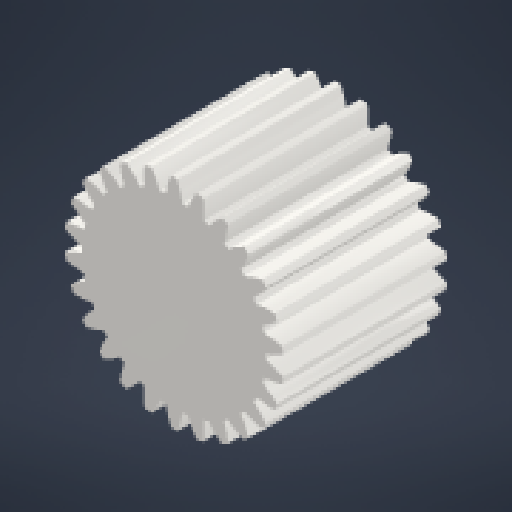
# Autodesk Inventor part: Цилиндрическое зубчатое зацепление1
Saved by Autodesk Inventor 2025 (Build 290162000, 162)
## iProperties
Created: 2025-01-15
Part Number: Цилиндрическое зубчатое зацепление1
Material: Steel
Document SubType Name: Modeling
Designer: Phantom
Categories: <?xml version="1.0" encoding="UTF-16"?> <MemberInstance><Categories><FamilyTemplate><FamilyTemplateParameter ValueType="xs:double" Id="1" ObjectReferenceKey="da_z" ObjectType="kUserParameterObject"/><FamilyTemplateParameter ValueType="xs:double" Id="2" ObjectReferenceKey="da_b" ObjectType="kUserParameterObject"/><FamilyTemplateParameter ValueType="xs:double" Id="3" ObjectReferenceKey="da_beta" ObjectType="kUserParameterObject"/><FamilyTemplateParameter ValueType="xs:double" Id="4" ObjectReferenceKey="da_da" ObjectType="kUserParameterObject"/><FamilyTemplateParameter ValueType="xs:double" Id="5" ObjectReferenceKey="da_aw" ObjectType="kUserParameterObject"/><FamilyTemplateParameter ValueType="xs:string" Id="6" ObjectReferenceKey="EAIAABAAAACIAQAAAAAAAIAAAAAAAAAA" ObjectType="83910656" SubObjectId="SurfaceGeometry"/></FamilyTemplate><ParamToTemplateMap><ParamToTemplate CategoryParameter="//CategoryParameter[@InternalName='046C89C9-8512-4d59-83FE-43B91F4F132A']" TemplateParameter="1"/><ParamToTemplate CategoryParameter="//CategoryParameter[@InternalName='2552DF32-E462-4b46-AEBF-C6C7768E72AC']" TemplateParameter="2"/><ParamToTemplate CategoryParameter="//CategoryParameter[@InternalName='C9EE641D-15FC-4fae-A226-E94C4372FDD7']" TemplateParameter="3"/><ParamToTemplate><ParamToTemplate CategoryParameter="//CategoryParameter[@InternalName='00B6519A-459B-49c7-AD84-2E56D39A5744']" ConstantValue="0.000000"/></ParamToTemplate><ParamToTemplate><ParamToTemplate CategoryParameter="//CategoryParameter[@InternalName='04B31F0E-C7A6-4894-AA32-9629BEFACF47']" ConstantValue="1.000000"/></ParamToTemplate><ParamToTemplate><ParamToTemplate CategoryParameter="//CategoryParameter[@InternalName='43CBEC2E-7847-49e7-A936-2F7889FCB2D9']" ConstantValue="0.250000"/></ParamToTemplate><ParamToTemplate><ParamToTemplate CategoryParameter="//CategoryParameter[@InternalName='B1EFC894-105D-4ebd-86BF-FA20ED196853']" ConstantValue="0.350000"/></ParamToTemplate><ParamToTemplate><ParamToTemplate CategoryParameter="//CategoryParameter[@InternalName='51175063-3D10-4879-93E8-6246FE8B403D']" ConstantValue="2060000000.000000"/></ParamToTemplate><ParamToTemplate><ParamToTemplate CategoryParameter="//CategoryParameter[@InternalName='A3A52E27-4454-46a9-B0BD-C932399B70AF']" ConstantValue="0.300000"/></ParamToTemplate><ParamToTemplate><ParamToTemplate CategoryParameter="//CategoryParameter[@InternalName='91B76062-C214-41d9-B1B9-14D2AB99603D']" ConstantValue="0.100000"/></ParamToTemplate><ParamToTemplate><ParamToTemplate CategoryParameter="//CategoryParameter[@InternalName='374E806E-8B8A-4dda-A9AA-1039D6500AD2']" ConstantValue="10.000000"/></ParamToTemplate><ParamToTemplate><ParamToTemplate CategoryParameter="//CategoryParameter[@InternalName='2D373A89-B862-43d6-8D0B-0CBF12AB9F6C']" ConstantValue="0.349066"/></ParamToTemplate><ParamToTemplate CategoryParameter="//CategoryParameter[@InternalName='37777632-D6A2-4fac-9D53-DB8ACD95C989']" TemplateParameter="4"/><ParamToTemplate CategoryParameter="//CategoryParameter[@InternalName='FD1017F1-B727-4f7e-9707-0F86F1FF9423']" TemplateParameter="5"/><ParamToTemplate><ParamToTemplate CategoryParameter="//CategoryParameter[@InternalName='9E1B4470-B2D3-4ff1-B813-535BB4CDF51A']" ConstantValue="3520000.000000"/></ParamToTemplate><ParamToTemplate><ParamToTemplate CategoryParameter="//CategoryParameter[@InternalName='F8452263-BFF6-458c-9FB1-07C4B99E95CD']" ConstantValue="11400000.000000"/></ParamToTemplate><ParamToTemplate><ParamToTemplate CategoryParameter="//CategoryParameter[@InternalName='3E3BB259-FD49-497f-8171-6EBC954A3479']" ConstantValue="2.000000"/></ParamToTemplate><ParamToTemplate CategoryParameter="//CategoryParameter[@InternalName='27C3BAF2-7550-4e4b-AE2C-0DB134B7D9B7']" TemplateParameter="6"/></ParamToTemplateMap><Category DisplayName="Gear" InternalName="DC85795E-93AB-48d5-8EEE-5A27447B64BD" Mnemonic="Gear"><CategoryParameter DisplayName="z" InternalName="046C89C9-8512-4d59-83FE-43B91F4F132A" Mnemonic="z"/><CategoryParameter DisplayName="b" InternalName="2552DF32-E462-4b46-AEBF-C6C7768E72AC" Mnemonic="b"/><CategoryParameter DisplayName="||b|" InternalName="C9EE641D-15FC-4fae-A226-E94C4372FDD7" Mnemonic="beta"/><CategoryParameter DisplayName="x" InternalName="00B6519A-459B-49c7-AD84-2E56D39A5744" Mnemonic="x"/><CategoryParameter DisplayName="a*" InternalName="04B31F0E-C7A6-4894-AA32-9629BEFACF47" Mnemonic="a"/><CategoryParameter DisplayName="c*" InternalName="43CBEC2E-7847-49e7-A936-2F7889FCB2D9" Mnemonic="c"/><CategoryParameter DisplayName="r|.f|*" InternalName="B1EFC894-105D-4ebd-86BF-FA20ED196853" Mnemonic="rf"/><CategoryParameter DisplayName="E" InternalName="51175063-3D10-4879-93E8-6246FE8B403D" Mnemonic="E"/><CategoryParameter DisplayName="||m|" InternalName="A3A52E27-4454-46a9-B0BD-C932399B70AF" Mnemonic="mi"/><Category DisplayName="SpurGear" InternalName="26C5A22E-A91E-4dfd-A3B3-23CCAFAE1764" Mnemonic="SpurGear"><CategoryParameter DisplayName="m" InternalName="91B76062-C214-41d9-B1B9-14D2AB99603D" Mnemonic="m"/><CategoryParameter DisplayName="P" InternalName="374E806E-8B8A-4dda-A9AA-1039D6500AD2" Mnemonic="PP"/><CategoryParameter DisplayName="||a|" InternalName="2D373A89-B862-43d6-8D0B-0CBF12AB9F6C" Mnemonic="alpha"/><CategoryParameter DisplayName="d|.a|" InternalName="37777632-D6A2-4fac-9D53-DB8ACD95C989" Mnemonic="da"/><CategoryParameter DisplayName="a|.w|" InternalName="FD1017F1-B727-4f7e-9707-0F86F1FF9423" Mnemonic="aw"/><CategoryParameter DisplayName="||s||.Flim|" InternalName="9E1B4470-B2D3-4ff1-B813-535BB4CDF51A" Mnemonic="sFlim"/><CategoryParameter DisplayName="||s||.Hlim|" InternalName="F8452263-BFF6-458c-9FB1-07C4B99E95CD" Mnemonic="sHlim"/><CategoryParameter DisplayName="тип" InternalName="3E3BB259-FD49-497f-8171-6EBC954A3479" Mnemonic="type"/><CategoryParameter DisplayName="PitchDiameter" InternalName="27C3BAF2-7550-4e4b-AE2C-0DB134B7D9B7" Mnemonic="IDS_PITCHDIAM"/></Category></Category></Categories></MemberInstance>
Density: 1 g/cm^3
Appearance: Steel
CustomPartVersion: 1
Author: Phantom
Autodesk Inventor part; units mm, degrees
ref_plane "YZ Plane" through (0, 0, 0) normal (1, 0, 0) x (0, 1, 0)
ref_plane "XZ Plane" through (0, 0, 0) normal (0, 1, 0) x (-1, 0, 0)
ref_plane "XY Plane" through (0, 0, 0) normal (0, 0, 1) x (1, 0, 0)
sketch "Sketch1" plane through (0, 0, 0) normal (0, 0, 1) x (1, 0, 0)
  circle A0 centre (0, 0) radius 12
  dimension "d0" = 24
  constraints: 1 centre point
  measures "d0" diameter of A0
extrude "Extrusion1" add sketch "Sketch1" along normal blind 20
ref_plane "Work Plane2" through (0, 0, 10) normal (0, 0, 1) x (1, 0, 0)
sketch "Sketch2" plane through (0, 0, 0) normal (0, 0, -1) x (-1, 0, 0)
  circle A0 centre (0, 0) radius 12 projected
  circle A1 centre (0, 0) radius 11
  dimension "d3" = 22
  constraints: 1 centre point, 1 coincident
  measures "d3" diameter of A1
surface extrude "Средний диаметр" sketch "Sketch2" against normal through all shown no curves A1
ref_plane "Work Plane8" through (0, 0, 0) normal (0.9898214, 0.1423148, 0) x (0, 0, 1)
ref_plane "Work Plane9" through (0, 0, 0) normal (1, 0, 0) x (0, 1, 0)
spur gear teeth "Цилиндрическое зубчатое зацепление" teeth 22 pitch diameter 22 tip diameter 24 root diameter 19.5 face width 20 start plane through (0, 0, 0) normal (0, 0, -1) x (-1, 0, 0)
sketch "Эскиз3" plane through (0, 0, 20) normal (0, 0, 1) x (1, 0, 0)
  arc A0 (-2.9677, 11.6272) -> (-3.7896, 11.3859) centre (0, 0) ccw projected
  arc A1 (-3.7896, 11.3859) -> (-3.7312, 9.0078) centre (4.8512, 10.4085) ccw projected
  arc A2 (-3.7312, 9.0078) -> (-4.3643, 8.7187) centre (0, 0) ccw projected
  arc A3 (-4.3643, 8.7187) -> (-6.1232, 10.3202) centre (-11.043, 3.1498) ccw projected
  arc A4 (-6.1232, 10.3202) -> (-6.8439, 9.857) centre (0, 0) ccw projected
  arc A5 (-6.8439, 9.857) -> (-6.1178, 7.5918) centre (1.7222, 11.3536) ccw projected
  arc A6 (-6.1178, 7.5918) -> (-6.6438, 7.136) centre (0, 0) ccw projected
  arc A7 (-6.6438, 7.136) -> (-8.7827, 8.177) centre (-11.4831, -0.0889) ccw projected
  arc A8 (-8.7827, 8.177) -> (-9.3437, 7.5296) centre (0, 0) ccw projected
  arc A9 (-9.3437, 7.5296) -> (-8.0089, 5.5606) centre (-1.5462, 11.3789) ccw projected
  arc A10 (-8.0089, 5.5606) -> (-8.3851, 4.9751) centre (0, 0) ccw projected
  arc A11 (-8.3851, 4.9751) -> (-10.7307, 5.3714) centre (-10.9929, -3.3205) ccw projected
  arc A12 (-10.7307, 5.3714) -> (-11.0866, 4.5922) centre (0, 0) ccw projected
  arc A13 (-11.0866, 4.5922) -> (-9.2511, 3.079) centre (-4.6894, 10.4823) ccw projected
  arc A14 (-9.2511, 3.079) -> (-9.4471, 2.4112) centre (0, 0) ccw projected
  arc A15 (-9.4471, 2.4112) -> (-11.8093, 2.1306) centre (-9.6121, -6.2831) ccw projected
  arc A16 (-11.8093, 2.1306) -> (-11.9312, 1.2827) centre (0, 0) ccw projected
  arc A17 (-11.9312, 1.2827) -> (-9.7438, 0.348) centre (-7.4526, 8.7366) ccw projected
  arc A18 (-9.7438, 0.348) -> (-9.7438, -0.348) centre (0, 0) ccw projected
  arc A19 (-9.7438, -0.348) -> (-11.9312, -1.2827) centre (-7.4526, -8.7366) ccw projected
  arc A20 (-11.9312, -1.2827) -> (-11.8093, -2.1306) centre (0, 0) ccw projected
  arc A21 (-11.8093, -2.1306) -> (-9.4471, -2.4112) centre (-9.6121, 6.2831) ccw projected
  arc A22 (-9.4471, -2.4112) -> (-9.2511, -3.079) centre (0, 0) ccw projected
  arc A23 (-9.2511, -3.079) -> (-11.0866, -4.5922) centre (-4.6894, -10.4823) ccw projected
  arc A24 (-11.0866, -4.5922) -> (-10.7307, -5.3714) centre (0, 0) ccw projected
  arc A25 (-10.7307, -5.3714) -> (-8.3851, -4.9751) centre (-10.9929, 3.3205) ccw projected
  arc A26 (-8.3851, -4.9751) -> (-8.0089, -5.5606) centre (0, 0) ccw projected
  arc A27 (-8.0089, -5.5606) -> (-9.3437, -7.5296) centre (-1.5462, -11.3789) ccw projected
  arc A28 (-9.3437, -7.5296) -> (-8.7827, -8.177) centre (0, 0) ccw projected
  arc A29 (-8.7827, -8.177) -> (-6.6438, -7.136) centre (-11.4831, 0.0889) ccw projected
  arc A30 (-6.6438, -7.136) -> (-6.1178, -7.5918) centre (0, 0) ccw projected
  arc A31 (-6.1178, -7.5918) -> (-6.8439, -9.857) centre (1.7222, -11.3536) ccw projected
  arc A32 (-6.8439, -9.857) -> (-6.1232, -10.3202) centre (0, 0) ccw projected
  arc A33 (-6.1232, -10.3202) -> (-4.3643, -8.7187) centre (-11.043, -3.1498) ccw projected
  arc A34 (-4.3643, -8.7187) -> (-3.7312, -9.0078) centre (0, 0) ccw projected
  arc A35 (-3.7312, -9.0078) -> (-3.7896, -11.3859) centre (4.8512, -10.4085) ccw projected
  arc A36 (-3.7896, -11.3859) -> (-2.9677, -11.6272) centre (0, 0) ccw projected
  arc A37 (-2.9677, -11.6272) -> (-1.7311, -9.5951) centre (-9.7083, -6.1334) ccw projected
  arc A38 (-1.7311, -9.5951) -> (-1.0422, -9.6941) centre (0, 0) ccw projected
  arc A39 (-1.0422, -9.6941) -> (-0.4283, -11.9924) centre (7.5871, -8.6201) ccw projected
  arc A40 (-0.4283, -11.9924) -> (0.4283, -11.9924) centre (0, 0) ccw projected
  arc A41 (0.4283, -11.9924) -> (1.0422, -9.6941) centre (-7.5871, -8.6201) ccw projected
  arc A42 (1.0422, -9.6941) -> (1.7311, -9.5951) centre (0, 0) ccw projected
  arc A43 (1.7311, -9.5951) -> (2.9677, -11.6272) centre (9.7083, -6.1334) ccw projected
  arc A44 (2.9677, -11.6272) -> (3.7896, -11.3859) centre (0, 0) ccw projected
  arc A45 (3.7896, -11.3859) -> (3.7312, -9.0078) centre (-4.8512, -10.4085) ccw projected
  arc A46 (3.7312, -9.0078) -> (4.3643, -8.7187) centre (0, 0) ccw projected
  arc A47 (4.3643, -8.7187) -> (6.1232, -10.3202) centre (11.043, -3.1498) ccw projected
  arc A48 (6.1232, -10.3202) -> (6.8439, -9.857) centre (0, 0) ccw projected
  arc A49 (6.8439, -9.857) -> (6.1178, -7.5918) centre (-1.7222, -11.3536) ccw projected
  arc A50 (6.1178, -7.5918) -> (6.6438, -7.136) centre (0, 0) ccw projected
  arc A51 (6.6438, -7.136) -> (8.7827, -8.177) centre (11.4831, 0.0889) ccw projected
  arc A52 (8.7827, -8.177) -> (9.3437, -7.5296) centre (0, 0) ccw projected
  arc A53 (9.3437, -7.5296) -> (8.0089, -5.5606) centre (1.5462, -11.3789) ccw projected
  arc A54 (8.0089, -5.5606) -> (8.3851, -4.9751) centre (0, 0) ccw projected
  arc A55 (8.3851, -4.9751) -> (10.7307, -5.3714) centre (10.9929, 3.3205) ccw projected
  arc A56 (10.7307, -5.3714) -> (11.0866, -4.5922) centre (0, 0) ccw projected
  arc A57 (11.0866, -4.5922) -> (9.2511, -3.079) centre (4.6894, -10.4823) ccw projected
  arc A58 (9.2511, -3.079) -> (9.4471, -2.4112) centre (0, 0) ccw projected
  arc A59 (9.4471, -2.4112) -> (11.8093, -2.1306) centre (9.6121, 6.2831) ccw projected
  arc A60 (11.8093, -2.1306) -> (11.9312, -1.2827) centre (0, 0) ccw projected
  arc A61 (11.9312, -1.2827) -> (9.7438, -0.348) centre (7.4526, -8.7366) ccw projected
  arc A62 (9.7438, -0.348) -> (9.7438, 0.348) centre (0, 0) ccw projected
  arc A63 (9.7438, 0.348) -> (11.9312, 1.2827) centre (7.4526, 8.7366) ccw projected
  arc A64 (11.9312, 1.2827) -> (11.8093, 2.1306) centre (0, 0) ccw projected
  arc A65 (11.8093, 2.1306) -> (9.4471, 2.4112) centre (9.6121, -6.2831) ccw projected
  arc A66 (9.4471, 2.4112) -> (9.2511, 3.079) centre (0, 0) ccw projected
  arc A67 (9.2511, 3.079) -> (11.0866, 4.5922) centre (4.6894, 10.4823) ccw projected
  arc A68 (11.0866, 4.5922) -> (10.7307, 5.3714) centre (0, 0) ccw projected
  arc A69 (10.7307, 5.3714) -> (8.3851, 4.9751) centre (10.9929, -3.3205) ccw projected
  arc A70 (8.3851, 4.9751) -> (8.0089, 5.5606) centre (0, 0) ccw projected
  arc A71 (8.0089, 5.5606) -> (9.3437, 7.5296) centre (1.5462, 11.3789) ccw projected
  arc A72 (9.3437, 7.5296) -> (8.7827, 8.177) centre (0, 0) ccw projected
  arc A73 (8.7827, 8.177) -> (6.6438, 7.136) centre (11.4831, -0.0889) ccw projected
  arc A74 (6.6438, 7.136) -> (6.1178, 7.5918) centre (0, 0) ccw projected
  arc A75 (6.1178, 7.5918) -> (6.8439, 9.857) centre (-1.7222, 11.3536) ccw projected
  arc A76 (6.8439, 9.857) -> (6.1232, 10.3202) centre (0, 0) ccw projected
  arc A77 (6.1232, 10.3202) -> (4.3643, 8.7187) centre (11.043, 3.1498) ccw projected
  arc A78 (4.3643, 8.7187) -> (3.7312, 9.0078) centre (0, 0) ccw projected
  arc A79 (3.7312, 9.0078) -> (3.7896, 11.3859) centre (-4.8512, 10.4085) ccw projected
  arc A80 (3.7896, 11.3859) -> (2.9677, 11.6272) centre (0, 0) ccw projected
  arc A81 (2.9677, 11.6272) -> (1.7311, 9.5951) centre (9.7083, 6.1334) ccw projected
  arc A82 (1.7311, 9.5951) -> (1.0422, 9.6941) centre (0, 0) ccw projected
  arc A83 (1.0422, 9.6941) -> (0.4283, 11.9924) centre (-7.5871, 8.6201) ccw projected
  arc A84 (0.4283, 11.9924) -> (-0.4283, 11.9924) centre (0, 0) ccw projected
  arc A85 (-0.4283, 11.9924) -> (-1.0422, 9.6941) centre (7.5871, 8.6201) ccw projected
  arc A86 (-1.0422, 9.6941) -> (-1.7311, 9.5951) centre (0, 0) ccw projected
  arc A87 (-1.7311, 9.5951) -> (-2.9677, 11.6272) centre (-9.7083, 6.1334) ccw projected
equation "\"d0\" = da_da"
equation "\"d1\" = da_b"
equation "\"d3\" = da_d"
equation "\"d16\" = da_aw"
equation "\"d43\" = da_aw"
equation "\"d46\" = da_aw"
equation "\"da_da\" = 24"
equation "\"da_b\" = 20"
equation "\"da_d\" = 22"
equation "\"da_aw\" = 26.5"
body "Solid1"
body "Srf1"
